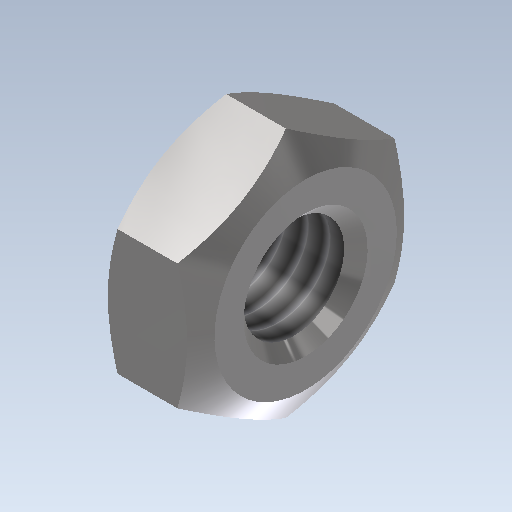
# Autodesk Inventor part: NTJ-010C
Saved by Autodesk Inventor 2021.3 (Build 253353010, 353A)
## iProperties
Created: 2019-10-24
Part Number: NTJ-010C
Material: ステンレス鋼
Catalog Web Link: www.cadenas.de
Description: CJ2-Z_NTJ-Rod End Nut
Vendor: SMC
Document SubType Name: Modeling
Designer: psadmin
Manufacturer: SMC
Mass: 0.80585 g
Surface Area: 1.58248 cm^2
Volume: 0.100731 cm^3
Density: 8 g/cm^3
Appearance: 半つや出し
Category: PARTsolutions
Company: SMC
PSOL_IDENT_0: {$CADENAS_DATA\23d-libs\smc_jp\actuator\standard_air_cylinder\cj2\accessories\cj2_z_ntj.prj},159 {VT
PSOL_IDENT_1: YP=3D},{NB=NTJ-010C},{LINA=NTJ-010C},{NN=CJ2-Z_NTJ},{DATE=07.02.2019 07:31:59},{GEOMDATE=04.05.2016
PSOL_IDENT_2: 08:42:11},{VERSION=},{LINEID=80},{WBVAR=},{WBNUMERIC=}  {NB=NTJ-010C},{LINA=NTJ-010C},{KT=DUMMY},{MO
PSOL_IDENT_3: DEL=NTJ-010C},{BORE=10},{B2=7.0},{C2=8.1},{D=M4x0.7},{D1=4},{D2=0.7},{H2=3.2},{DW=5.88}
NN: CJ2-Z_NTJ
NT: Rod End Nut
NB: NTJ-010C
NBSYN: $MODEL.
LINA: NTJ-010C
MODEL: NTJ-010C
BORE: 10
B2: 7
C2: 8.1
D: M4x0.7
H2: 3.2
SUPPLIER: SMC
ARTICLENO: NTJ-010C
BOMINFO: NTJ-010C
CREATOR: CADENAS GmbH
Title: NTJ-010C
Author: Cadenas PARTsolutions
Comments: Rod End Nut
Autodesk Inventor part; units mm, degrees
sketch "B" plane through (0, 0, 0) normal (1, 0, 0) x (0, 1, 0)
  line L0 (-2.0207, 3.5) -> (-4.0415, 0)
  line L1 (-4.0415, 0) -> (-2.0207, -3.5)
  line L2 (-2.0207, -3.5) -> (2.0207, -3.5)
  line L3 (2.0207, -3.5) -> (4.0415, 0)
  line L4 (4.0415, 0) -> (2.0207, 3.5)
  line L5 (2.0207, 3.5) -> (-2.0207, 3.5)
  constraints: 12 end point
extrude "Extrusion1" add sketch "B" along normal mid plane 3.2
sketch "Sketch_2" plane through (0, 0, 0) normal (0, 0, 1) x (1, 0, 0)
  line L0 (1.6, 0) -> (-1.6, 0)
  line L1 (-1.6, 0) -> (-1.6, 2)
  line L2 (-1.6, 2) -> (-1.221, 1.621)
  line L3 (-1.221, 1.621) -> (1.221, 1.621)
  line L4 (1.221, 1.621) -> (1.6, 2)
  line L5 (1.6, 2) -> (1.6, 0)
  line L6 (1.6, 0) -> (-1.6, 0)
  constraints: 14 end point
revolve "Revolution1" cut sketch "Sketch_2" angle 360 about axis through (1.6, 0, 0) along (1, 0, 0)
thread "Thread1" size "M4x0.7" class "6H" standard "ISO Metric profile" full length
sketch "Sketch_3" plane through (0, 0, 0) normal (0, 0, 1) x (1, 0, 0)
  line L0 (50, 0) -> (-50, 0)
  line L1 (-6.6, 6.94) -> (-6.6, 1)
  line L2 (-6.6, 1) -> (-1.6, 1)
  line L3 (-1.6, 1) -> (-1.6, 2.94)
  line L4 (-1.6, 2.94) -> (0, 5.7113)
  line L5 (0, 5.7113) -> (1.6, 2.94)
  line L6 (1.6, 2.94) -> (1.6, 1)
  line L7 (1.6, 1) -> (6.6, 1)
  line L8 (6.6, 1) -> (6.6, 6.94)
  line L9 (6.6, 6.94) -> (-6.6, 6.94)
  constraints: 20 end point
revolve "Revolution2" cut sketch "Sketch_3" angle 360 about axis through (50, 0, 0) along (1, 0, 0)
ref_plane "nt_XY" through (0, 0, 0) normal (1, 0, 0) x (0, 0, -1)
ref_plane "nt_YZ" through (0, 0, 0) normal (0, 0, -1) x (0, 1, 0)
ref_plane "nt_ZX" through (0, 0, 0) normal (0, 1, 0) x (1, 0, 0)
ref_plane "ntj_XY" through (1.6, 0, 0) normal (1, 0, 0) x (0, 0, -1)
ref_plane "ntj_YZ" through (1.6, 0, 0) normal (0, 0, -1) x (0, 1, 0)
ref_plane "ntj_ZX" through (1.6, 0, 0) normal (0, 1, 0) x (1, 0, 0)
body "Solid1"
